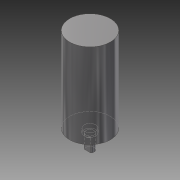
# Autodesk Inventor part: Motor
Saved by Autodesk Inventor 2015 (Build 190159000, 159)
## iProperties
Created: 2014-07-28
Part Number: Motor
Material: Stainless Steel
Document SubType Name: Modeling
Designer: karl
Density: 8 g/cm^3
Appearance: Semi-Polished
Author: karl
Autodesk Inventor part; units mm, degrees
ref_plane "YZ Plane" through (0, 0, 0) normal (1, 0, 0) x (0, 1, 0)
ref_plane "XZ Plane" through (0, 0, 0) normal (0, 1, 0) x (-1, 0, 0)
ref_plane "XY Plane" through (0, 0, 0) normal (0, 0, 1) x (1, 0, 0)
sketch "Sketch1" plane through (0, 0, 0) normal (0, 0, 1) x (1, 0, 0)
  circle A0 centre (0, 0) radius 12.5
  dimension "d0" = 25
  constraints: 1 centre point, 1 coincident
  measures "d0" diameter of A0
extrude "Extrusion1" add sketch "Sketch1" along normal blind 52
sketch "Sketch2" plane through (0, 0, 0) normal (0, 0, -1) x (-1, 0, 0)
  circle A0 centre (0, 0) radius 3.5
  dimension "d3" = 7
  constraints: 1 centre point, 1 coincident
  measures "d3" diameter of A0
extrude "Extrusion2" add sketch "Sketch2" along normal blind 2.5
sketch "Sketch3" plane through (0, 0, -2.5) normal (0, 0, -1) x (-1, 0, 0)
  circle A0 centre (0, 0) radius 2.5
  dimension "d6" = 5
  constraints: 1 centre point, 1 coincident
  measures "d6" diameter of A0
extrude "Extrusion3" add sketch "Sketch3" along normal blind 9
sketch "Sketch4" plane through (0, 0, -11.5) normal (0, 0, -1) x (-1, 0, 0)
  line L0 (2, -1.5) -> (-2, -1.5)
  circle A0 centre (0, 0) radius 2.5 projected
  dimension "d9" = 1.5
  constraints: 2 end point, 2 point on circle, 1 horizontal
  measures "d9" distance from line of point (0, 0) L0
extrude "Extrusion4" cut sketch "Sketch4" against normal blind 8 contours A0 L0 picked at (-0.534, -1.6398)
sketch "Sketch5" plane through (0, 0, 0) normal (0, 0, -1) x (-1, 0, 0)
  circle A0 centre (0, -8.5) radius 1.5
  circle A1 centre (0, 8.5) radius 1.5
  point P0 (0, 0)
  dimension "d12" = 3
  dimension "d13" = 8.5
  dimension "d14" = 3
  dimension "d15" = 17
  constraints: 2 centre point, 2 vertical alignment
  measures "d12" diameter of A0
  measures "d13" distance of A0.centre point (0, 0)
  measures "d14" diameter of A1
  measures "d15" distance of A0.centre A1.centre
extrude "Extrusion5" cut sketch "Sketch5" against normal blind 3
body "Solid1"
